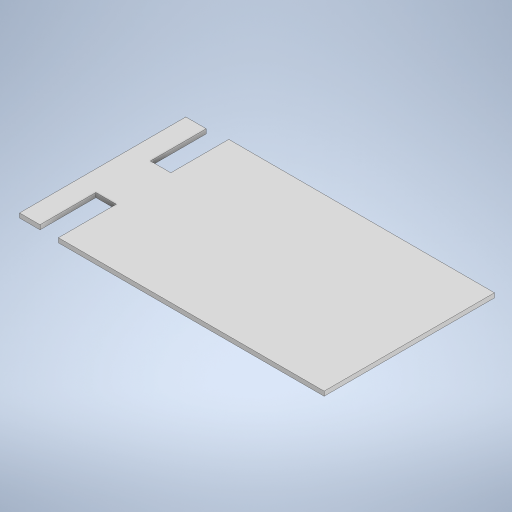
# Autodesk Inventor part: suelo_imp
Saved by Autodesk Inventor 2024 (Build 280153000, 153)
## iProperties
Created: 2023-05-01
Part Number: suelo_imp
Material: Generic
Document SubType Name: Modeling
Designer: Diego
Density: 1 g/cm^3
Appearance: Default
Author: Diego
Autodesk Inventor part; units mm, degrees
ref_plane "YZ Plane" through (0, 0, 0) normal (1, 0, 0) x (0, 1, 0)
ref_plane "XZ Plane" through (0, 0, 0) normal (0, 1, 0) x (-1, 0, 0)
ref_plane "XY Plane" through (0, 0, 0) normal (0, 0, 1) x (1, 0, 0)
sketch "Sketch1" plane through (0, 0, 0) normal (0, 1, 0) x (-1, 0, 0)
  line L0 (-97.5, -62.5) -> (97.5, -62.5)
  line L1 (97.5, 62.5) -> (-97.5, 62.5)
  line L2 (-97.5, 62.5) -> (-97.5, -62.5)
  line L3 (-97.5, -62.5) -> (97.5, 62.5) construction
  line L4 (97.5, -62.5) -> (-97.5, 62.5) construction
  line L5 (97.5, 20) -> (112.5, 20)
  line L6 (127.5, 20) -> (127.5, -20)
  line L7 (112.5, -20) -> (97.5, -20)
  line L8 (97.5, -62.5) -> (97.5, -20)
  line L9 (97.5, 20) -> (97.5, 62.5)
  line L10 (112.5, 20) -> (112.5, 61)
  line L11 (112.5, 61) -> (127.5, 61)
  line L12 (127.5, 61) -> (127.5, 20)
  line L13 (127.5, 0) -> (97.5, 0) construction
  line L14 (112.5, -20) -> (112.5, -61)
  line L15 (112.5, -61) -> (127.5, -61)
  line L16 (127.5, -61) -> (127.5, -20)
  point P0 (0, 0)
  dimension "d0" = 195
  dimension "d1" = 125
  dimension "d3" = 30
  dimension "d4" = 40
  dimension "d5" = 15
  dimension "d6" = 41
  dimension "d7" = 15
  dimension "d8" = 1.5
  constraints: 34 end point, 8 perpendicular, 3 horizontal, 3 midpoint, 3 parallel, 3 symmetric about line
  measures "d0" distance of L1.end L1.start
  measures "d1" distance of L1.start L0.end
  measures "d3" distance of L5.start L6.start
  measures "d4" distance of L6.start L6.end
  measures "d5" distance of L5.end L6.start
  measures "d6" distance of L5.end L10.end
  measures "d7" distance between parallel lines of L10 L6
  measures "d8" distance between parallel lines of L11 L1
extrude "Extrusion1" add sketch "Sketch1" along normal blind 3.25
body "Solid1"
